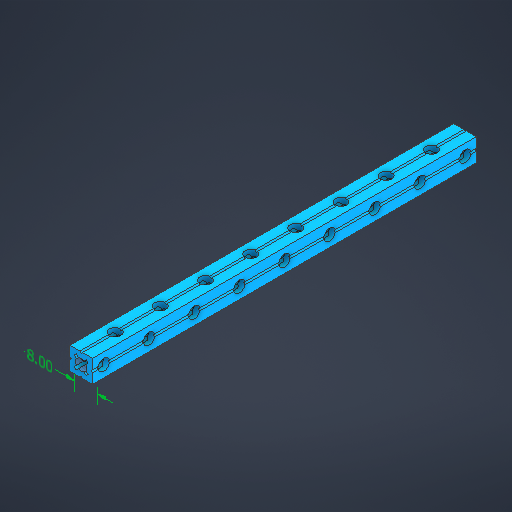
# Autodesk Inventor part: Beam9x8x1-136
Saved by Autodesk Inventor 2026.1 (Build 301233020, 233B)
## iProperties
Created: 2025-10-11
Part Number: Beam9x8x1-136
Material: Generic
Document SubType Name: Modeling
Designer: Asus
Density: 1 g/cm^3
Appearance: Default
Author: Asus
Autodesk Inventor part; units mm, degrees
ref_plane "YZ Plane" through (0, 0, 0) normal (1, 0, 0) x (0, 1, 0)
ref_plane "XZ Plane" through (0, 0, 0) normal (0, 1, 0) x (-1, 0, 0)
ref_plane "XY Plane" through (0, 0, 0) normal (0, 0, 1) x (1, 0, 0)
sketch "Sketch1" plane through (0, 0, 0) normal (0, 0, 1) x (1, 0, 0)
  line L0 (-1.6663, 4) -> (10.9416, 4) construction
  line L1 (0, 0) -> (8, 8) construction
  line L2 (0, 8) -> (8, 0) construction
  line L3 (4, 9.5924) -> (4, 6) construction
  line L4 (4, 4) -> (4, -1.2867) construction
  arc A0 (2.2771, 5.0158) -> (2.2771, 2.9842) centre (4, 4) ccw
  arc A1 (5.0158, 5.7229) -> (2.9842, 5.7229) centre (4, 4) ccw
  arc A2 (2.9842, 2.2771) -> (5.0158, 2.2771) centre (4, 4) ccw
  arc A3 (5.7229, 2.9842) -> (5.7229, 5.0158) centre (4, 4) ccw
  line L5 (2.2322, 6.4749) -> (1.5251, 5.7678)
  line L6 (4, 7.5355) -> (4.4645, 8)
  line L7 (4, 7.5355) -> (3.5355, 8)
  line L8 (6.4749, 2.2322) -> (5.7678, 1.5251)
  line L9 (1.57, 2.2771) -> (2.2771, 1.57)
  line L10 (5.7229, 6.43) -> (6.43, 5.7229)
  line L11 (7.5355, 4) -> (8, 4.4645)
  line L12 (7.5355, 4) -> (8, 3.5355)
  line L13 (4, 0.4645) -> (4.4645, 0)
  line L14 (4, 0.4645) -> (3.5355, 0)
  line L15 (0.4645, 4) -> (0, 3.5355)
  line L16 (0.4645, 4) -> (0, 4.4645)
  line L17 (8, 0) -> (8, 3.5355)
  line L18 (8, 4.4645) -> (8, 8)
  line L19 (8, 8) -> (4.4645, 8)
  line L20 (3.5355, 8) -> (0, 8)
  line L21 (0, 8) -> (0, 4.4645)
  line L22 (0, 3.5355) -> (0, 0)
  line L23 (0, 0) -> (3.5355, 0)
  line L24 (4.4645, 0) -> (8, 0)
  line L25 (5.7229, 5.0158) -> (6.43, 5.7229)
  line L26 (5.7229, 6.43) -> (5.0158, 5.7229)
  line L27 (2.9842, 5.7229) -> (2.2322, 6.4749)
  line L28 (1.5251, 5.7678) -> (2.2771, 5.0158)
  line L29 (2.2771, 2.9842) -> (1.57, 2.2771)
  line L30 (2.2771, 1.57) -> (2.9842, 2.2771)
  line L31 (5.0158, 2.2771) -> (5.7678, 1.5251)
  line L32 (6.4749, 2.2322) -> (5.7229, 2.9842)
  point P0 (5.7678, 5.7678)
  point P1 (5.9221, 5.215)
  point P2 (1.577, 1.577)
  point P3 (4, 7.1371)
  point P4 (7.1371, 4)
  point P5 (4, 0.8629)
  point P6 (0.8629, 4)
  dimension "d0" = 8
  dimension "d1" = 8
  dimension "d27" = 1
  dimension "d31" = 1
  constraints: 66 end point, 18 parallel, 15 point on line, 9 point on circle, 7 perpendicular, 4 centre point, 3 horizontal, 2 midpoint, 2 vertical
  measures "d0" distance of L2.start L1.end
  measures "d1" distance of L1.end L2.end
  measures "d27" distance of L8.start L8.end
  measures "d31" distance of L10.start L10.end
extrude "Extrusion1" add sketch "Sketch1" against normal blind 136 contours L28 L5 L27 A1 L26 L10 L25 A3 L32 L8 L31 A2 L30 L9 L29 A0 | L6 L19 L18 L11 L12 L17 L24 L13 L14 L23 L22 L15 L16 L21 L20 L7
sketch "Sketch2" plane through (0, 0, 0) normal (1, 0, 0) x (0, 1, 0)
  line L0 (4, 0) -> (4, -136) construction
  circle A0 centre (4, -4.03) radius 2
  circle A1 centre (4, -20.03) radius 2
  circle A2 centre (4, -36.03) radius 2
  circle A3 centre (4, -52.03) radius 2
  circle A4 centre (4, -68.03) radius 2
  circle A5 centre (4, -84.03) radius 2
  circle A6 centre (4, -100.03) radius 2
  circle A7 centre (4, -116.03) radius 2
  circle A8 centre (4, -132.03) radius 2
  point P0 (0, 0)
  dimension "d14" = 4
  dimension "d15" = 4.03
  dimension "d18" = 16
  constraints: 9 centre point, 1 point on line, 1 vertical, 16 other
  measures "d14" diameter of A0
  measures "d15" distance of L0.start A0.centre
  measures "d18" distance of A0.centre A1.centre
extrude "Extrusion2" cut sketch "Sketch2" along normal blind 136
sketch "Sketch3" plane through (0, 0, 0) normal (0, 0, 1) x (1, 0, 0)
  line L0 (-1.6701, 4) -> (10.9379, 4) construction
  line L1 (0, 0) -> (8, 8) construction
  line L2 (0, 8) -> (8, 0) construction
  line L3 (4, 9.5781) -> (4, 5.9857) construction
  line L4 (4, 4) -> (4, -1.3011) construction
  arc A0 (2.2765, 5.0161) -> (2.2752, 2.9862) centre (4, 4) ccw
  arc A1 (5.0085, 5.7105) -> (2.9915, 5.7105) centre (4, 4) ccw
  arc A2 (2.9898, 2.2866) -> (5.005, 2.2835) centre (4, 4) ccw
  arc A3 (5.7121, 2.9906) -> (5.7156, 5.0034) centre (4, 4) ccw
  line L5 (2.2211, 6.4809) -> (1.5164, 5.7762)
  line L6 (4, 7.5355) -> (4.4645, 8)
  line L7 (4, 7.5355) -> (3.5355, 8)
  line L8 (6.4641, 2.2386) -> (5.757, 1.5315)
  line L9 (1.4685, 2.1795) -> (2.1756, 1.4724)
  line L10 (5.7156, 6.4176) -> (6.4227, 5.7105)
  line L11 (7.5355, 4) -> (8, 4.4645)
  line L12 (7.5355, 4) -> (8, 3.5355)
  line L13 (4, 0.4645) -> (4.4645, 0)
  line L14 (4, 0.4645) -> (3.5355, 0)
  line L15 (0.4645, 4) -> (0, 3.5355)
  line L16 (0.4645, 4) -> (0, 4.4645)
  line L17 (8, 0) -> (8, 3.5355)
  line L18 (8, 4.4645) -> (8, 8)
  line L19 (8, 8) -> (4.4645, 8)
  line L20 (3.5355, 8) -> (0, 8)
  line L21 (0, 8) -> (0, 4.4645)
  line L22 (0, 3.5355) -> (0, 0)
  line L23 (0, 0) -> (3.5355, 0)
  line L24 (4.4645, 0) -> (8, 0)
  line L25 (5.7156, 5.0034) -> (6.4227, 5.7105)
  line L26 (5.7156, 6.4176) -> (5.0085, 5.7105)
  line L27 (2.9915, 5.7105) -> (2.2211, 6.4809)
  line L28 (1.5164, 5.7762) -> (2.2765, 5.0161)
  line L29 (2.2752, 2.9862) -> (1.4685, 2.1795)
  line L30 (2.1756, 1.4724) -> (2.9898, 2.2866)
  line L31 (5.005, 2.2835) -> (5.757, 1.5315)
  line L32 (6.4641, 2.2386) -> (5.7121, 2.9906)
  point P0 (5.7587, 5.7587)
  point P1 (5.9183, 5.2007)
  point P2 (1.568, 1.568)
  point P3 (4, 7.1228)
  point P4 (7.1333, 4)
  point P5 (4, 0.8486)
  point P6 (0.8592, 4)
  point P7 (4, 4)
  dimension "d32" = 8
  dimension "d33" = 8
  dimension "d34" = 1
  dimension "d35" = 1
  dimension "d36" = 4
  dimension "d37" = 4
  dimension "d38" = 90
  dimension "d39" = 6
  dimension "d40" = 6
  dimension "d41" = 1
  dimension "d42" = 1
  constraints: 66 end point, 18 parallel, 14 point on line, 9 coincident, 9 point on circle, 7 perpendicular, 4 centre point, 3 horizontal, 3 midpoint, 2 vertical
  measures "d32" distance of L2.start L1.end
  measures "d33" distance of L1.end L2.end
  measures "d34" distance of L8.start L8.end
  measures "d35" distance of L10.start L10.end
  measures "d36" distance from line of L19 point (4, 4)
  measures "d37" distance from line of L22 point (4, 4)
  measures "d38" angle of L5 L27
  measures "d39" distance between parallel lines of L8 L5
  measures "d40" distance between parallel lines of L9 L10
  measures "d41" distance between parallel lines of L30 L29
  measures "d42" distance between parallel lines of L25 L26
extrude "Extrusion3" cut sketch "Sketch3" against normal blind 136 contours L28 L5 L27 A1 L26 L10 L25 A3 L32 L8 L31 A2 L30 L9 L29 A0
sketch "Sketch4" plane through (4.4645, 8, 0) normal (0, 1, 0) x (1, 0, 0)
  circle A0 centre (-0.4645, 12.03) radius 2
  line L0 (-0.4645, 0) -> (0, 0) projected
  line L1 (-0.4645, 136) -> (0, 136) projected
  line L2 (-0.4645, 0) -> (-0.4645, 136)
  circle A1 centre (-0.4645, 28.03) radius 2
  circle A2 centre (-0.4645, 44.03) radius 2
  circle A3 centre (-0.4645, 60.03) radius 2
  circle A4 centre (-0.4645, 76.03) radius 2
  circle A5 centre (-0.4645, 92.03) radius 2
  circle A6 centre (-0.4645, 108.03) radius 2
  circle A7 centre (-0.4645, 124.03) radius 2
  point P0 (-4.4645, 0)
  point P1 (-0.4645, 12.03)
  dimension "d45" = 4
  dimension "d48" = 16
  constraints: 8 centre point, 2 end point, 2 vertical, 1 coincident, 14 other
  measures "d45" diameter of A0
  measures "d48" distance of A0.centre A1.centre
extrude "Extrusion4" cut sketch "Sketch4" against normal blind 10
thread "Thread1" size "M4x0.7" class "6H" standard "ANSI Metric M Profile" full length
thread "Thread2" size "M4x0.7" class "6H" standard "ANSI Metric M Profile" full length
thread "Thread3" size "M4x0.7" class "6H" standard "ANSI Metric M Profile" full length
thread "Thread4" size "M4x0.7" class "6H" standard "ANSI Metric M Profile" full length
body "Solid1"
